Autodesk Fusion 360 part; units mm, degrees
(part 2 of 4)
  line L926 (106.594, 72.9326) -> (106.594, 69.8334)
  line L927 (106.594, 69.8334) -> (107.395, 69.8334)
  line L928 (107.395, 69.8334) -> (107.395, 64.0334)
  line L929 (107.395, 64.0334) -> (106.594, 64.0334)
  line L930 (106.594, 64.0334) -> (106.594, 60.9328)
  line L931 (106.594, 60.9328) -> (107.395, 60.9328)
  line L932 (107.395, 60.9328) -> (107.395, 59.9338)
  line L933 (107.395, 59.9338) -> (121.394, 59.9338)
  line L934 (121.394, 59.9338) -> (121.394, 60.9328)
  line L935 (121.394, 60.9328) -> (122.195, 60.9328)
  line L936 (122.195, 60.9328) -> (122.195, 64.0334)
  line L937 (122.195, 64.0334) -> (121.394, 64.0334)
  line L938 (121.394, 64.0334) -> (121.394, 69.8334)
  line L939 (121.394, 69.8334) -> (122.195, 69.8334)
  line L940 (122.195, 69.8334) -> (122.195, 72.9326)
  line L941 (122.195, 72.9326) -> (121.394, 72.9326)
  line L942 (121.394, 72.9326) -> (121.394, 73.9331)
  line L943 (121.394, 73.9331) -> (107.395, 73.9331)
  line L944 (126.445, 73.9331) -> (126.445, 72.9326)
  line L945 (126.445, 72.9326) -> (125.644, 72.9326)
  line L946 (125.644, 72.9326) -> (125.644, 69.8334)
  line L947 (125.644, 69.8334) -> (126.445, 69.8334)
  line L948 (126.445, 69.8334) -> (126.445, 64.0334)
  line L949 (126.445, 64.0334) -> (125.644, 64.0334)
  line L950 (125.644, 64.0334) -> (125.644, 60.9328)
  line L951 (125.644, 60.9328) -> (126.445, 60.9328)
  line L952 (126.445, 60.9328) -> (126.445, 59.9338)
  line L953 (126.445, 59.9338) -> (140.444, 59.9338)
  line L954 (140.444, 59.9338) -> (140.444, 60.9328)
  line L955 (140.444, 60.9328) -> (141.245, 60.9328)
  line L956 (141.245, 60.9328) -> (141.245, 64.0334)
  line L957 (141.245, 64.0334) -> (140.444, 64.0334)
  line L958 (140.444, 64.0334) -> (140.444, 69.8334)
  line L959 (140.444, 69.8334) -> (141.245, 69.8334)
  line L960 (141.245, 69.8334) -> (141.245, 72.9326)
  line L961 (141.245, 72.9326) -> (140.444, 72.9326)
  line L962 (140.444, 72.9326) -> (140.444, 73.9331)
  line L963 (140.444, 73.9331) -> (126.445, 73.9331)
  line L964 (145.495, 73.9331) -> (145.495, 72.9326)
  line L965 (145.495, 72.9326) -> (144.694, 72.9326)
  line L966 (144.694, 72.9326) -> (144.694, 69.8334)
  line L967 (144.694, 69.8334) -> (145.495, 69.8334)
  line L968 (145.495, 69.8334) -> (145.495, 64.0334)
  line L969 (145.495, 64.0334) -> (144.694, 64.0334)
  line L970 (144.694, 64.0334) -> (144.694, 60.9328)
  line L971 (144.694, 60.9328) -> (145.495, 60.9328)
  line L972 (145.495, 60.9328) -> (145.495, 59.9338)
  line L973 (145.495, 59.9338) -> (159.494, 59.9338)
  line L974 (159.494, 59.9338) -> (159.494, 60.9328)
  line L975 (159.494, 60.9328) -> (160.295, 60.9328)
  line L976 (160.295, 60.9328) -> (160.295, 64.0334)
  line L977 (160.295, 64.0334) -> (159.494, 64.0334)
  line L978 (159.494, 64.0334) -> (159.494, 69.8334)
  line L979 (159.494, 69.8334) -> (160.295, 69.8334)
  line L980 (160.295, 69.8334) -> (160.295, 72.9326)
  line L981 (160.295, 72.9326) -> (159.494, 72.9326)
  line L982 (159.494, 72.9326) -> (159.494, 73.9331)
  line L983 (159.494, 73.9331) -> (145.495, 73.9331)
  line L984 (164.545, 73.9331) -> (164.545, 72.9326)
  line L985 (164.545, 72.9326) -> (163.744, 72.9326)
  line L986 (163.744, 72.9326) -> (163.744, 69.8334)
  line L987 (163.744, 69.8334) -> (164.545, 69.8334)
  line L988 (164.545, 69.8334) -> (164.545, 64.0334)
  line L989 (164.545, 64.0334) -> (163.744, 64.0334)
  line L990 (163.744, 64.0334) -> (163.744, 60.9328)
  line L991 (163.744, 60.9328) -> (164.545, 60.9328)
  line L992 (164.545, 60.9328) -> (164.545, 59.9338)
  line L993 (164.545, 59.9338) -> (178.544, 59.9338)
  line L994 (178.544, 59.9338) -> (178.544, 60.9328)
  line L995 (178.544, 60.9328) -> (179.345, 60.9328)
  line L996 (179.345, 60.9328) -> (179.345, 64.0334)
  line L997 (179.345, 64.0334) -> (178.544, 64.0334)
  line L998 (178.544, 64.0334) -> (178.544, 69.8334)
  line L999 (178.544, 69.8334) -> (179.345, 69.8334)
  line L1000 (179.345, 69.8334) -> (179.345, 72.9326)
  line L1001 (179.345, 72.9326) -> (178.544, 72.9326)
  line L1002 (178.544, 72.9326) -> (178.544, 73.9331)
  line L1003 (178.544, 73.9331) -> (164.545, 73.9331)
  line L1004 (183.595, 73.9331) -> (183.595, 72.9326)
  line L1005 (183.595, 72.9326) -> (182.794, 72.9326)
  line L1006 (182.794, 72.9326) -> (182.794, 69.8334)
  line L1007 (182.794, 69.8334) -> (183.595, 69.8334)
  line L1008 (183.595, 69.8334) -> (183.595, 64.0334)
  line L1009 (183.595, 64.0334) -> (182.794, 64.0334)
  line L1010 (182.794, 64.0334) -> (182.794, 60.9328)
  line L1011 (182.794, 60.9328) -> (183.595, 60.9328)
  line L1012 (183.595, 60.9328) -> (183.595, 59.9338)
  line L1013 (183.595, 59.9338) -> (197.594, 59.9338)
  line L1014 (197.594, 59.9338) -> (197.594, 60.9328)
  line L1015 (197.594, 60.9328) -> (198.395, 60.9328)
  line L1016 (198.395, 60.9328) -> (198.395, 64.0334)
  line L1017 (198.395, 64.0334) -> (197.594, 64.0334)
  line L1018 (197.594, 64.0334) -> (197.594, 69.8334)
  line L1019 (197.594, 69.8334) -> (198.395, 69.8334)
  line L1020 (198.395, 69.8334) -> (198.395, 72.9326)
  line L1021 (198.395, 72.9326) -> (197.594, 72.9326)
  line L1022 (197.594, 72.9326) -> (197.594, 73.9331)
  line L1023 (197.594, 73.9331) -> (183.595, 73.9331)
  line L1024 (202.645, 73.9331) -> (202.645, 72.9326)
  line L1025 (202.645, 72.9326) -> (201.844, 72.9326)
  line L1026 (201.844, 72.9326) -> (201.844, 69.8334)
  line L1027 (201.844, 69.8334) -> (202.645, 69.8334)
  line L1028 (202.645, 69.8334) -> (202.645, 64.0334)
  line L1029 (202.645, 64.0334) -> (201.844, 64.0334)
  line L1030 (201.844, 64.0334) -> (201.844, 60.9328)
  line L1031 (201.844, 60.9328) -> (202.645, 60.9328)
  line L1032 (202.645, 60.9328) -> (202.645, 59.9338)
  line L1033 (202.645, 59.9338) -> (216.644, 59.9338)
  line L1034 (216.644, 59.9338) -> (216.644, 60.9328)
  line L1035 (216.644, 60.9328) -> (217.445, 60.9328)
  line L1036 (217.445, 60.9328) -> (217.445, 64.0334)
  line L1037 (217.445, 64.0334) -> (216.644, 64.0334)
  line L1038 (216.644, 64.0334) -> (216.644, 69.8334)
  line L1039 (216.644, 69.8334) -> (217.445, 69.8334)
  line L1040 (217.445, 69.8334) -> (217.445, 72.9326)
  line L1041 (217.445, 72.9326) -> (216.644, 72.9326)
  line L1042 (216.644, 72.9326) -> (216.644, 73.9331)
  line L1043 (216.644, 73.9331) -> (202.645, 73.9331)
  line L1044 (221.695, 73.9331) -> (221.695, 72.9326)
  line L1045 (221.695, 72.9326) -> (220.894, 72.9326)
  line L1046 (220.894, 72.9326) -> (220.894, 69.8334)
  line L1047 (220.894, 69.8334) -> (221.695, 69.8334)
  line L1048 (221.695, 69.8334) -> (221.695, 64.0334)
  line L1049 (221.695, 64.0334) -> (220.894, 64.0334)
  line L1050 (220.894, 64.0334) -> (220.894, 60.9328)
  line L1051 (220.894, 60.9328) -> (221.695, 60.9328)
  line L1052 (221.695, 60.9328) -> (221.695, 59.9338)
  line L1053 (221.695, 59.9338) -> (235.694, 59.9338)
  line L1054 (235.694, 59.9338) -> (235.694, 60.9328)
  line L1055 (235.694, 60.9328) -> (236.495, 60.9328)
  line L1056 (236.495, 60.9328) -> (236.495, 64.0334)
  line L1057 (236.495, 64.0334) -> (235.694, 64.0334)
  line L1058 (235.694, 64.0334) -> (235.694, 69.8334)
  line L1059 (235.694, 69.8334) -> (236.495, 69.8334)
  line L1060 (236.495, 69.8334) -> (236.495, 72.9326)
  line L1061 (236.495, 72.9326) -> (235.694, 72.9326)
  line L1062 (235.694, 72.9326) -> (235.694, 73.9331)
  line L1063 (235.694, 73.9331) -> (221.695, 73.9331)
  line L1064 (240.745, 73.9331) -> (240.745, 72.9326)
  line L1065 (240.745, 72.9326) -> (239.944, 72.9326)
  line L1066 (239.944, 72.9326) -> (239.944, 69.8334)
  line L1067 (239.944, 69.8334) -> (240.745, 69.8334)
  line L1068 (240.745, 69.8334) -> (240.745, 64.0334)
  line L1069 (240.745, 64.0334) -> (239.944, 64.0334)
  line L1070 (239.944, 64.0334) -> (239.944, 60.9328)
  line L1071 (239.944, 60.9328) -> (240.745, 60.9328)
  line L1072 (240.745, 60.9328) -> (240.745, 59.9338)
  line L1073 (240.745, 59.9338) -> (254.744, 59.9338)
  line L1074 (254.744, 59.9338) -> (254.744, 60.9328)
  line L1075 (254.744, 60.9328) -> (255.545, 60.9328)
  line L1076 (255.545, 60.9328) -> (255.545, 64.0334)
  line L1077 (255.545, 64.0334) -> (254.744, 64.0334)
  line L1078 (254.744, 64.0334) -> (254.744, 69.8334)
  line L1079 (254.744, 69.8334) -> (255.545, 69.8334)
  line L1080 (255.545, 69.8334) -> (255.545, 72.9326)
  line L1081 (255.545, 72.9326) -> (254.744, 72.9326)
  line L1082 (254.744, 72.9326) -> (254.744, 73.9331)
  line L1083 (254.744, 73.9331) -> (240.745, 73.9331)
  line L1084 (264.557, 73.9331) -> (264.557, 72.9326)
  line L1085 (264.557, 72.9326) -> (263.756, 72.9326)
  line L1086 (263.756, 72.9326) -> (263.756, 69.8334)
  line L1087 (263.756, 69.8334) -> (264.557, 69.8334)
  line L1088 (264.557, 69.8334) -> (264.557, 64.0334)
  line L1089 (264.557, 64.0334) -> (263.756, 64.0334)
  line L1090 (263.756, 64.0334) -> (263.756, 60.9328)
  line L1091 (263.756, 60.9328) -> (264.557, 60.9328)
  line L1092 (264.557, 60.9328) -> (264.557, 59.9338)
  line L1093 (264.557, 59.9338) -> (278.557, 59.9338)
  line L1094 (278.557, 59.9338) -> (278.557, 60.9328)
  line L1095 (278.557, 60.9328) -> (279.356, 60.9328)
  line L1096 (279.356, 60.9328) -> (279.356, 64.0334)
  line L1097 (279.356, 64.0334) -> (278.557, 64.0334)
  line L1098 (278.557, 64.0334) -> (278.557, 69.8334)
  line L1099 (278.557, 69.8334) -> (279.356, 69.8334)
  line L1100 (279.356, 69.8334) -> (279.356, 72.9326)
  line L1101 (279.356, 72.9326) -> (278.557, 72.9326)
  line L1102 (278.557, 72.9326) -> (278.557, 73.9331)
  line L1103 (278.557, 73.9331) -> (264.557, 73.9331)
  line L1104 (259.795, 92.9831) -> (259.795, 91.9826)
  line L1105 (259.795, 91.9826) -> (258.994, 91.9826)
  line L1106 (258.994, 91.9826) -> (258.994, 88.8834)
  line L1107 (258.994, 88.8834) -> (259.795, 88.8834)
  line L1108 (259.795, 88.8834) -> (259.795, 88.2826)
  line L1109 (259.795, 88.2826) -> (258.269, 88.2826)
  line L1110 (258.269, 88.2826) -> (258.269, 91.5127)
  line L1111 (258.269, 91.5127) -> (256.544, 91.5127)
  line L1112 (256.544, 91.5127) -> (256.544, 92.4348)
  line L1113 (256.544, 92.4348) -> (253.243, 92.4348)
  line L1114 (253.243, 92.4348) -> (253.243, 91.5127)
  line L1115 (253.243, 91.5127) -> (251.52, 91.5127)
  line L1116 (251.52, 91.5127) -> (251.52, 88.2826)
  line L1117 (251.52, 88.2826) -> (250.694, 88.2826)
  line L1118 (250.694, 88.2826) -> (250.694, 85.4837)
  line L1119 (250.694, 85.4837) -> (251.52, 85.4837)
  line L1120 (251.52, 85.4837) -> (251.52, 79.2138)
  line L1121 (251.52, 79.2138) -> (253.243, 79.2138)
  line L1122 (253.243, 79.2138) -> (253.243, 78.2327)
  line L1123 (253.243, 78.2327) -> (256.544, 78.2327)
  line L1124 (256.544, 78.2327) -> (256.544, 79.2138)
  line L1125 (256.544, 79.2138) -> (258.269, 79.2138)
  line L1126 (258.269, 79.2138) -> (258.269, 83.6828)
  line L1127 (258.269, 83.6828) -> (259.795, 83.6828)
  line L1128 (259.795, 83.6828) -> (259.795, 83.0834)
  line L1129 (259.795, 83.0834) -> (258.994, 83.0834)
  line L1130 (258.994, 83.0834) -> (258.994, 79.9828)
  line L1131 (258.994, 79.9828) -> (259.795, 79.9828)
  line L1132 (259.795, 79.9828) -> (259.795, 78.9838)
  line L1133 (259.795, 78.9838) -> (273.794, 78.9838)
  line L1134 (273.794, 78.9838) -> (273.794, 79.9828)
  line L1135 (273.794, 79.9828) -> (274.595, 79.9828)
  line L1136 (274.595, 79.9828) -> (274.595, 83.0834)
  line L1137 (274.595, 83.0834) -> (273.794, 83.0834)
  line L1138 (273.794, 83.0834) -> (273.794, 83.6828)
  line L1139 (273.794, 83.6828) -> (275.32, 83.6828)
  line L1140 (275.32, 83.6828) -> (275.32, 79.2138)
  line L1141 (275.32, 79.2138) -> (277.045, 79.2138)
  line L1142 (277.045, 79.2138) -> (277.045, 78.2327)
  line L1143 (277.045, 78.2327) -> (280.344, 78.2327)
  line L1144 (280.344, 78.2327) -> (280.344, 79.2138)
  line L1145 (280.344, 79.2138) -> (282.069, 79.2138)
  line L1146 (282.069, 79.2138) -> (282.069, 85.4837)
  line L1147 (282.069, 85.4837) -> (282.895, 85.4837)
  line L1148 (282.895, 85.4837) -> (282.895, 88.2826)
  line L1149 (282.895, 88.2826) -> (282.069, 88.2826)
  line L1150 (282.069, 88.2826) -> (282.069, 91.5127)
  line L1151 (282.069, 91.5127) -> (280.344, 91.5127)
  line L1152 (280.344, 91.5127) -> (280.344, 92.4348)
  line L1153 (280.344, 92.4348) -> (277.045, 92.4348)
  line L1154 (277.045, 92.4348) -> (277.045, 91.5127)
  line L1155 (277.045, 91.5127) -> (275.32, 91.5127)
  line L1156 (275.32, 91.5127) -> (275.32, 88.2826)
  line L1157 (275.32, 88.2826) -> (273.794, 88.2826)
  line L1158 (273.794, 88.2826) -> (273.794, 88.8834)
  line L1159 (273.794, 88.8834) -> (274.595, 88.8834)
  line L1160 (274.595, 88.8834) -> (274.595, 91.9826)
  line L1161 (274.595, 91.9826) -> (273.794, 91.9826)
  line L1162 (273.794, 91.9826) -> (273.794, 92.9831)
  line L1163 (273.794, 92.9831) -> (259.795, 92.9831)
  line L1164 (2.6197, 92.9831) -> (2.6197, 91.9826)
  line L1165 (2.6197, 91.9826) -> (1.819, 91.9826)
  line L1166 (1.819, 91.9826) -> (1.819, 88.8834)
  line L1167 (1.819, 88.8834) -> (2.6197, 88.8834)
  line L1168 (2.6197, 88.8834) -> (2.6197, 83.0834)
  line L1169 (2.6197, 83.0834) -> (1.819, 83.0834)
  line L1170 (1.819, 83.0834) -> (1.819, 79.9828)
  line L1171 (1.819, 79.9828) -> (2.6197, 79.9828)
  line L1172 (2.6197, 79.9828) -> (2.6197, 78.9838)
  line L1173 (2.6197, 78.9838) -> (16.6192, 78.9838)
  line L1174 (16.6192, 78.9838) -> (16.6192, 79.9828)
  line L1175 (16.6192, 79.9828) -> (17.4198, 79.9828)
  line L1176 (17.4198, 79.9828) -> (17.4198, 83.0834)
  line L1177 (17.4198, 83.0834) -> (16.6192, 83.0834)
  line L1178 (16.6192, 83.0834) -> (16.6192, 88.8834)
  line L1179 (16.6192, 88.8834) -> (17.4198, 88.8834)
  line L1180 (17.4198, 88.8834) -> (17.4198, 91.9826)
  line L1181 (17.4198, 91.9826) -> (16.6192, 91.9826)
  line L1182 (16.6192, 91.9826) -> (16.6192, 92.9831)
  line L1183 (16.6192, 92.9831) -> (2.6196, 92.9831)
  line L1184 (21.6697, 92.9831) -> (21.6697, 91.9826)
  line L1185 (21.6697, 91.9826) -> (20.869, 91.9826)
  line L1186 (20.869, 91.9826) -> (20.869, 88.8834)
  line L1187 (20.869, 88.8834) -> (21.6697, 88.8834)
  line L1188 (21.6697, 88.8834) -> (21.6697, 83.0834)
  line L1189 (21.6697, 83.0834) -> (20.869, 83.0834)
  line L1190 (20.869, 83.0834) -> (20.869, 79.9828)
  line L1191 (20.869, 79.9828) -> (21.6697, 79.9828)
  line L1192 (21.6697, 79.9828) -> (21.6697, 78.9838)
  line L1193 (21.6697, 78.9838) -> (35.669, 78.9838)
  line L1194 (35.669, 78.9838) -> (35.669, 79.9828)
  line L1195 (35.669, 79.9828) -> (36.4698, 79.9828)
  line L1196 (36.4698, 79.9828) -> (36.4698, 83.0834)
  line L1197 (36.4698, 83.0834) -> (35.669, 83.0834)
  line L1198 (35.669, 83.0834) -> (35.669, 88.8834)
  line L1199 (35.669, 88.8834) -> (36.4698, 88.8834)
  line L1200 (36.4698, 88.8834) -> (36.4698, 91.9826)
  line L1201 (36.4698, 91.9826) -> (35.669, 91.9826)
  line L1202 (35.669, 91.9826) -> (35.669, 92.9831)
  line L1203 (35.669, 92.9831) -> (21.6697, 92.9831)
  line L1204 (40.7197, 92.9831) -> (40.7197, 91.9826)
  line L1205 (40.7197, 91.9826) -> (39.9189, 91.9826)
  line L1206 (39.9189, 91.9826) -> (39.9189, 88.8834)
  line L1207 (39.9189, 88.8834) -> (40.7197, 88.8834)
  line L1208 (40.7197, 88.8834) -> (40.7197, 83.0834)
  line L1209 (40.7197, 83.0834) -> (39.9189, 83.0834)
  line L1210 (39.9189, 83.0834) -> (39.9189, 79.9828)
  line L1211 (39.9189, 79.9828) -> (40.7197, 79.9828)
  line L1212 (40.7197, 79.9828) -> (40.7197, 78.9838)
  line L1213 (40.7197, 78.9838) -> (54.719, 78.9838)
  line L1214 (54.719, 78.9838) -> (54.719, 79.9828)
  line L1215 (54.719, 79.9828) -> (55.5198, 79.9828)
  line L1216 (55.5198, 79.9828) -> (55.5198, 83.0834)
  line L1217 (55.5198, 83.0834) -> (54.719, 83.0834)
  line L1218 (54.719, 83.0834) -> (54.719, 88.8834)
  line L1219 (54.719, 88.8834) -> (55.5198, 88.8834)
  line L1220 (55.5198, 88.8834) -> (55.5198, 91.9826)
  line L1221 (55.5198, 91.9826) -> (54.719, 91.9826)
  line L1222 (54.719, 91.9826) -> (54.719, 92.9831)
  line L1223 (54.719, 92.9831) -> (40.7197, 92.9831)
  line L1224 (59.7697, 92.9831) -> (59.7697, 91.9826)
  line L1225 (59.7697, 91.9826) -> (58.9689, 91.9826)
  line L1226 (58.9689, 91.9826) -> (58.9689, 88.8834)
  line L1227 (58.9689, 88.8834) -> (59.7697, 88.8834)
  line L1228 (59.7697, 88.8834) -> (59.7697, 83.0834)
  line L1229 (59.7697, 83.0834) -> (58.9689, 83.0834)
  line L1230 (58.9689, 83.0834) -> (58.9689, 79.9828)
  line L1231 (58.9689, 79.9828) -> (59.7697, 79.9828)
  line L1232 (59.7697, 79.9828) -> (59.7697, 78.9838)
  line L1233 (59.7697, 78.9838) -> (73.769, 78.9838)
  line L1234 (73.769, 78.9838) -> (73.769, 79.9828)
  line L1235 (73.769, 79.9828) -> (74.5698, 79.9828)
  line L1236 (74.5698, 79.9828) -> (74.5698, 83.0834)
  line L1237 (74.5698, 83.0834) -> (73.769, 83.0834)
  line L1238 (73.769, 83.0834) -> (73.769, 88.8834)
  line L1239 (73.769, 88.8834) -> (74.5698, 88.8834)
  line L1240 (74.5698, 88.8834) -> (74.5698, 91.9826)
  line L1241 (74.5698, 91.9826) -> (73.769, 91.9826)
  line L1242 (73.769, 91.9826) -> (73.769, 92.9831)
  line L1243 (73.769, 92.9831) -> (59.7697, 92.9831)
  line L1244 (78.8197, 92.9831) -> (78.8197, 91.9826)
  line L1245 (78.8197, 91.9826) -> (78.0189, 91.9826)
  line L1246 (78.0189, 91.9826) -> (78.0189, 88.8834)
  line L1247 (78.0189, 88.8834) -> (78.8197, 88.8834)
  line L1248 (78.8197, 88.8834) -> (78.8197, 83.0834)
  line L1249 (78.8197, 83.0834) -> (78.0189, 83.0834)
  line L1250 (78.0189, 83.0834) -> (78.0189, 79.9828)
  line L1251 (78.0189, 79.9828) -> (78.8197, 79.9828)
  line L1252 (78.8197, 79.9828) -> (78.8197, 78.9838)
  line L1253 (78.8197, 78.9838) -> (92.819, 78.9838)
  line L1254 (92.819, 78.9838) -> (92.819, 79.9828)
  line L1255 (92.819, 79.9828) -> (93.6184, 79.9828)
  line L1256 (93.6184, 79.9828) -> (93.6184, 83.0834)
  line L1257 (93.6184, 83.0834) -> (92.819, 83.0834)
  line L1258 (92.819, 83.0834) -> (92.819, 88.8834)
  line L1259 (92.819, 88.8834) -> (93.6184, 88.8834)
  line L1260 (93.6184, 88.8834) -> (93.6184, 91.9826)
  line L1261 (93.6184, 91.9826) -> (92.819, 91.9826)
  line L1262 (92.819, 91.9826) -> (92.819, 92.9831)
  line L1263 (92.819, 92.9831) -> (78.8197, 92.9831)
  line L1264 (97.8683, 92.9831) -> (97.8683, 91.9826)
  line L1265 (97.8683, 91.9826) -> (97.0689, 91.9826)
  line L1266 (97.0689, 91.9826) -> (97.0689, 88.8834)
  line L1267 (97.0689, 88.8834) -> (97.8683, 88.8834)
  line L1268 (97.8683, 88.8834) -> (97.8683, 83.0834)
  line L1269 (97.8683, 83.0834) -> (97.0689, 83.0834)
  line L1270 (97.0689, 83.0834) -> (97.0689, 79.9828)
  line L1271 (97.0689, 79.9828) -> (97.8683, 79.9828)
  line L1272 (97.8683, 79.9828) -> (97.8683, 78.9838)
  line L1273 (97.8683, 78.9838) -> (111.869, 78.9838)
  line L1274 (111.869, 78.9838) -> (111.869, 79.9828)
  line L1275 (111.869, 79.9828) -> (112.668, 79.9828)
  line L1276 (112.668, 79.9828) -> (112.668, 83.0834)
  line L1277 (112.668, 83.0834) -> (111.869, 83.0834)
  line L1278 (111.869, 83.0834) -> (111.869, 88.8834)
  line L1279 (111.869, 88.8834) -> (112.668, 88.8834)
  line L1280 (112.668, 88.8834) -> (112.668, 91.9826)
  line L1281 (112.668, 91.9826) -> (111.869, 91.9826)
  line L1282 (111.869, 91.9826) -> (111.869, 92.9831)
  line L1283 (111.869, 92.9831) -> (97.8683, 92.9831)
  line L1284 (116.918, 92.9831) -> (116.918, 91.9826)
  line L1285 (116.918, 91.9826) -> (116.119, 91.9826)
  line L1286 (116.119, 91.9826) -> (116.119, 88.8834)
  line L1287 (116.119, 88.8834) -> (116.918, 88.8834)
  line L1288 (116.918, 88.8834) -> (116.918, 83.0834)
  line L1289 (116.918, 83.0834) -> (116.119, 83.0834)
  line L1290 (116.119, 83.0834) -> (116.119, 79.9828)
  line L1291 (116.119, 79.9828) -> (116.918, 79.9828)
  line L1292 (116.918, 79.9828) -> (116.918, 78.9838)
  line L1293 (116.918, 78.9838) -> (130.919, 78.9838)
  line L1294 (130.919, 78.9838) -> (130.919, 79.9828)
  line L1295 (130.919, 79.9828) -> (131.72, 79.9828)
  line L1296 (131.72, 79.9828) -> (131.72, 83.0834)
  line L1297 (131.72, 83.0834) -> (130.919, 83.0834)
  line L1298 (130.919, 83.0834) -> (130.919, 88.8834)
  line L1299 (130.919, 88.8834) -> (131.72, 88.8834)
  line L1300 (131.72, 88.8834) -> (131.72, 91.9826)
  line L1301 (131.72, 91.9826) -> (130.919, 91.9826)
  line L1302 (130.919, 91.9826) -> (130.919, 92.9831)
  line L1303 (130.919, 92.9831) -> (116.918, 92.9831)
  line L1304 (135.97, 92.9831) -> (135.97, 91.9826)
  line L1305 (135.97, 91.9826) -> (135.169, 91.9826)
  line L1306 (135.169, 91.9826) -> (135.169, 88.8834)
  line L1307 (135.169, 88.8834) -> (135.97, 88.8834)
  line L1308 (135.97, 88.8834) -> (135.97, 83.0834)
  line L1309 (135.97, 83.0834) -> (135.169, 83.0834)
  line L1310 (135.169, 83.0834) -> (135.169, 79.9828)
  line L1311 (135.169, 79.9828) -> (135.97, 79.9828)
  line L1312 (135.97, 79.9828) -> (135.97, 78.9838)
  line L1313 (135.97, 78.9838) -> (149.969, 78.9838)
  line L1314 (149.969, 78.9838) -> (149.969, 79.9828)
  line L1315 (149.969, 79.9828) -> (150.77, 79.9828)
  line L1316 (150.77, 79.9828) -> (150.77, 83.0834)
  line L1317 (150.77, 83.0834) -> (149.969, 83.0834)
  line L1318 (149.969, 83.0834) -> (149.969, 88.8834)
  line L1319 (149.969, 88.8834) -> (150.77, 88.8834)
  line L1320 (150.77, 88.8834) -> (150.77, 91.9826)
  line L1321 (150.77, 91.9826) -> (149.969, 91.9826)
  line L1322 (149.969, 91.9826) -> (149.969, 92.9831)
  line L1323 (149.969, 92.9831) -> (135.97, 92.9831)
  line L1324 (155.02, 92.9831) -> (155.02, 91.9826)
  line L1325 (155.02, 91.9826) -> (154.219, 91.9826)
  line L1326 (154.219, 91.9826) -> (154.219, 88.8834)
  line L1327 (154.219, 88.8834) -> (155.02, 88.8834)
  line L1328 (155.02, 88.8834) -> (155.02, 83.0834)
  line L1329 (155.02, 83.0834) -> (154.219, 83.0834)
  line L1330 (154.219, 83.0834) -> (154.219, 79.9828)
  line L1331 (154.219, 79.9828) -> (155.02, 79.9828)
  line L1332 (155.02, 79.9828) -> (155.02, 78.9838)
  line L1333 (155.02, 78.9838) -> (169.019, 78.9838)
  line L1334 (169.019, 78.9838) -> (169.019, 79.9828)
  line L1335 (169.019, 79.9828) -> (169.82, 79.9828)
  line L1336 (169.82, 79.9828) -> (169.82, 83.0834)
  line L1337 (169.82, 83.0834) -> (169.019, 83.0834)
  line L1338 (169.019, 83.0834) -> (169.019, 88.8834)
  line L1339 (169.019, 88.8834) -> (169.82, 88.8834)
  line L1340 (169.82, 88.8834) -> (169.82, 91.9826)
  line L1341 (169.82, 91.9826) -> (169.019, 91.9826)
  line L1342 (169.019, 91.9826) -> (169.019, 92.9831)
  line L1343 (169.019, 92.9831) -> (155.02, 92.9831)
  line L1344 (174.07, 92.9831) -> (174.07, 91.9826)
  line L1345 (174.07, 91.9826) -> (173.269, 91.9826)
  line L1346 (173.269, 91.9826) -> (173.269, 88.8834)
  line L1347 (173.269, 88.8834) -> (174.07, 88.8834)
  line L1348 (174.07, 88.8834) -> (174.07, 83.0834)
  line L1349 (174.07, 83.0834) -> (173.269, 83.0834)
  line L1350 (173.269, 83.0834) -> (173.269, 79.9828)
  line L1351 (173.269, 79.9828) -> (174.07, 79.9828)
  line L1352 (174.07, 79.9828) -> (174.07, 78.9838)
  line L1353 (174.07, 78.9838) -> (188.069, 78.9838)
  line L1354 (188.069, 78.9838) -> (188.069, 79.9828)
  line L1355 (188.069, 79.9828) -> (188.87, 79.9828)
  line L1356 (188.87, 79.9828) -> (188.87, 83.0834)
  line L1357 (188.87, 83.0834) -> (188.069, 83.0834)
  line L1358 (188.069, 83.0834) -> (188.069, 88.8834)
  line L1359 (188.069, 88.8834) -> (188.87, 88.8834)
  line L1360 (188.87, 88.8834) -> (188.87, 91.9826)
  line L1361 (188.87, 91.9826) -> (188.069, 91.9826)
  line L1362 (188.069, 91.9826) -> (188.069, 92.9831)
  line L1363 (188.069, 92.9831) -> (174.07, 92.9831)
  line L1364 (193.12, 92.9831) -> (193.12, 91.9826)
  line L1365 (193.12, 91.9826) -> (192.319, 91.9826)
  line L1366 (192.319, 91.9826) -> (192.319, 88.8834)
  line L1367 (192.319, 88.8834) -> (193.12, 88.8834)
  line L1368 (193.12, 88.8834) -> (193.12, 83.0834)
  line L1369 (193.12, 83.0834) -> (192.319, 83.0834)
  line L1370 (192.319, 83.0834) -> (192.319, 79.9828)
  line L1371 (192.319, 79.9828) -> (193.12, 79.9828)
  line L1372 (193.12, 79.9828) -> (193.12, 78.9838)
  line L1373 (193.12, 78.9838) -> (207.119, 78.9838)
  line L1374 (207.119, 78.9838) -> (207.119, 79.9828)
  line L1375 (207.119, 79.9828) -> (207.92, 79.9828)
  line L1376 (207.92, 79.9828) -> (207.92, 83.0834)
  line L1377 (207.92, 83.0834) -> (207.119, 83.0834)
  line L1378 (207.119, 83.0834) -> (207.119, 88.8834)
  line L1379 (207.119, 88.8834) -> (207.92, 88.8834)
  line L1380 (207.92, 88.8834) -> (207.92, 91.9826)
  line L1381 (207.92, 91.9826) -> (207.119, 91.9826)
  line L1382 (207.119, 91.9826) -> (207.119, 92.9831)
  line L1383 (207.119, 92.9831) -> (193.12, 92.9831)
  line L1384 (212.17, 92.9831) -> (212.17, 91.9826)
  line L1385 (212.17, 91.9826) -> (211.369, 91.9826)
  line L1386 (211.369, 91.9826) -> (211.369, 88.8834)
  line L1387 (211.369, 88.8834) -> (212.17, 88.8834)
  line L1388 (212.17, 88.8834) -> (212.17, 83.0834)
  line L1389 (212.17, 83.0834) -> (211.369, 83.0834)
  line L1390 (211.369, 83.0834) -> (211.369, 79.9828)
  line L1391 (211.369, 79.9828) -> (212.17, 79.9828)
  line L1392 (212.17, 79.9828) -> (212.17, 78.9838)
  line L1393 (212.17, 78.9838) -> (226.169, 78.9838)
  line L1394 (226.169, 78.9838) -> (226.169, 79.9828)
  line L1395 (226.169, 79.9828) -> (226.97, 79.9828)
  line L1396 (226.97, 79.9828) -> (226.97, 83.0834)
  line L1397 (226.97, 83.0834) -> (226.169, 83.0834)
  line L1398 (226.169, 83.0834) -> (226.169, 88.8834)
  line L1399 (226.169, 88.8834) -> (226.97, 88.8834)
  line L1400 (226.97, 88.8834) -> (226.97, 91.9826)
  line L1401 (226.97, 91.9826) -> (226.169, 91.9826)
  line L1402 (226.169, 91.9826) -> (226.169, 92.9831)
  line L1403 (226.169, 92.9831) -> (212.17, 92.9831)
  line L1404 (231.22, 92.9831) -> (231.22, 91.9826)
  line L1405 (231.22, 91.9826) -> (230.419, 91.9826)
  line L1406 (230.419, 91.9826) -> (230.419, 88.8834)
  line L1407 (230.419, 88.8834) -> (231.22, 88.8834)
  line L1408 (231.22, 88.8834) -> (231.22, 83.0834)
  line L1409 (231.22, 83.0834) -> (230.419, 83.0834)
  line L1410 (230.419, 83.0834) -> (230.419, 79.9828)
  line L1411 (230.419, 79.9828) -> (231.22, 79.9828)
  line L1412 (231.22, 79.9828) -> (231.22, 78.9838)
  line L1413 (231.22, 78.9838) -> (245.219, 78.9838)
  line L1414 (245.219, 78.9838) -> (245.219, 79.9828)
  line L1415 (245.219, 79.9828) -> (246.02, 79.9828)
  line L1416 (246.02, 79.9828) -> (246.02, 83.0834)
  line L1417 (246.02, 83.0834) -> (245.219, 83.0834)
  line L1418 (245.219, 83.0834) -> (245.219, 88.8834)
  line L1419 (245.219, 88.8834) -> (246.02, 88.8834)
  line L1420 (246.02, 88.8834) -> (246.02, 91.9826)
  line L1421 (246.02, 91.9826) -> (245.219, 91.9826)
  line L1422 (245.219, 91.9826) -> (245.219, 92.9831)
  line L1423 (245.219, 92.9831) -> (231.22, 92.9831)
extrude "Extrude3" add sketch "48cd8e48e3c34c88b59e201f8eb7611360cf066c_switch" along normal blind 1.6 separate body makes body 2
move_body "Move1" bodies 2 to x (1, 0, 0) y (0, 1, 0) z (0, 0, 1) at (15, 9, -15)
extrude "Extrude4" add 1 faces at (205.595, 10.0667, -15.2577) along direction (0, 0, 1) blind 3 on bodies 2 bodies 2
extrude "Extrude5" add 1 faces at (205.595, 10.0667, -12.2577) along direction (0, 0, 1) blind 9 on bodies 2 bodies 2
extrude "Extrude6" add 1 faces at (15.0951, 9.5333, -74.7576) along direction (-1, 0, 0) blind 7 on bodies 2 bodies 2
extrude "Extrude7" add 1 faces at (105.6784, 9.5333, -3.2577) along direction (0, 0, 1) blind 1.3 on bodies 2 bodies 2
extrude "Extrude8" add 1 faces at (8.0951, 10.0667, -38.141) along direction (-1, 0, 0) blind 6.093 on bodies 2 bodies 2
fillet "Fillet7" radius 10 1 edges at (2.0021, 9.8, -1.9577) on bodies 2
extrude "Extrude9" add 1 faces at (201.2307, 9.5333, -110.5075) along direction (0, 0, -1) blind 38.45 on bodies 2 bodies 2
fillet "Fillet8" radius 10 1 edges at (2.0021, 9.8, -148.9575) on bodies 2
extrude "Extrude10" add 1 faces at (300.845, 9.5333, -50.9576) along direction (1, 0, 0) blind 7.1 on bodies 2 bodies 2
fillet "Fillet9" radius 10 1 edges at (307.945, 9.8, -1.9577) on bodies 2
fillet "Fillet10" radius 10 1 edges at (307.945, 9.8, -148.9575) on bodies 2
fillet "Fillet11" radius 3 8 edges at (2.9289, 14, -2.9289) (155, 14, 0) (307.0711, 14, -2.9289) (310, 14, -75.4964) (307.0711, 14, -148.0638) (155, 14, -150.9928) (2.9289, 14, -148.0638) (0, 14, -75.4964) on bodies 1
fillet "Fillet12" radius 0.5 16 edges at (307.9403, 14, -10.9088) (305.0711, 14, -4.9289) (299.0912, 14, -2.0597) (155, 14, -2) (10.9088, 14, -2.0597) (4.9289, 14, -4.9289) (2.0597, 14, -10.9088) (2, 14, -75.4964) (2.0597, 14, -140.0839) (4.9289, 14, -146.0638) (10.9088, 14, -148.9331) (155, 14, -148.9928) (299.0912, 14, -148.9331) (305.0711, 14, -146.0638) (307.9403, 14, -140.0839) (308, 14, -75.4964) on bodies 1
sketch "Sketch3" plane through (0, 0, 0) normal (-1, 0, 0) x (0, 0, 1)
  spline S0 degree 3 poles (-140.9928, 11.1033) (-140.3266, 11.1422) (-139.6599, 11.1716) (-138.9928, 11.1716) knots 4.126797 4.126797 4.126797 4.126797 4.326935 4.326935 4.326935 4.326935
  line L0 (-140.9928, 11.1033) -> (-140.9928, 0)
  line L1 (-140.9928, 0) -> (-10, 0)
  line L2 (-10, 0) -> (-10, 11.1033)
  spline S1 degree 3 poles (-12, 11.1716) (-11.333, 11.1716) (-10.666, 11.1422) (-10, 11.1033) knots 4.127933 4.127933 4.127933 4.127933 4.32807 4.32807 4.32807 4.32807
  line L3 (-12, 11.1716) -> (-138.9928, 11.1716)
  line L4 (-129.2, 9.2) -> (-129.2, 7.5)
  line L5 (-129.2, 7.5) -> (-128, 6.2)
  line L6 (-128, 6.2) -> (-122.3, 6.2)
  line L7 (-122.3, 6.2) -> (-121.1, 7.6)
  line L8 (-121.1, 7.6) -> (-121.1, 9.2)
  line L9 (-121.1, 9.2) -> (-129.2, 9.2)
  constraint perpendicular L3 L4
  constraint horizontal L6
  constraint perpendicular L6 L8
  constraint perpendicular L4 L9
extrude "Extrude11" cut sketch "Sketch3" against normal blind 11 contours L4 L5 L6 L7 L8 L9 bodies 1
sketch "Sketch4" plane through (0, 10.6, 0) normal (0, 1, 0) x (-1, 0, 0)
  arc A0 (-307.945, -138.9575) -> (-297.945, -148.9575) centre (-297.945, -138.9575) ccw
  line L0 (-297.945, -148.9575) -> (-12.0021, -148.9575)
  arc A1 (-12.0021, -148.9575) -> (-2.0021, -138.9575) centre (-12.0021, -138.9575) ccw
  line L1 (-2.0021, -138.9575) -> (-2.0021, -11.9577)
  arc A2 (-2.0021, -11.9577) -> (-12.0021, -1.9577) centre (-12.0021, -11.9577) ccw
  line L2 (-12.0021, -1.9577) -> (-297.945, -1.9577)
  arc A3 (-297.945, -1.9577) -> (-307.945, -11.9577) centre (-297.945, -11.9577) ccw
  line L3 (-307.945, -11.9577) -> (-307.945, -138.9575)
  line L4 (-236.695, -88.9331) -> (-250.694, -88.9331)
  line L5 (-250.694, -88.9331) -> (-250.694, -87.9326)
  line L6 (-250.694, -87.9326) -> (-251.495, -87.9326)
  line L7 (-251.495, -87.9326) -> (-251.495, -84.8334)
  line L8 (-251.495, -84.8334) -> (-250.694, -84.8334)
  line L9 (-250.694, -84.8334) -> (-250.694, -79.0334)
  line L10 (-250.694, -79.0334) -> (-251.495, -79.0334)
  line L11 (-251.495, -79.0334) -> (-251.495, -75.9328)
  line L12 (-251.495, -75.9328) -> (-250.694, -75.9328)
  line L13 (-250.694, -75.9328) -> (-250.694, -74.9338)
  line L14 (-250.694, -74.9338) -> (-236.695, -74.9338)
  line L15 (-236.695, -74.9338) -> (-236.695, -75.9328)
  line L16 (-236.695, -75.9328) -> (-235.894, -75.9328)
  line L17 (-235.894, -75.9328) -> (-235.894, -79.0334)
  line L18 (-235.894, -79.0334) -> (-236.695, -79.0334)
  line L19 (-236.695, -79.0334) -> (-236.695, -84.8334)
  line L20 (-236.695, -84.8334) -> (-235.894, -84.8334)
  line L21 (-235.894, -84.8334) -> (-235.894, -87.9326)
  line L22 (-235.894, -87.9326) -> (-236.695, -87.9326)
  line L23 (-236.695, -87.9326) -> (-236.695, -88.9331)
  line L24 (-255.745, -88.9331) -> (-269.744, -88.9331)
  line L25 (-269.744, -88.9331) -> (-269.744, -87.9326)
  line L26 (-269.744, -87.9326) -> (-270.545, -87.9326)
  line L27 (-270.545, -87.9326) -> (-270.545, -84.8334)
  line L28 (-270.545, -84.8334) -> (-269.744, -84.8334)
  line L29 (-269.744, -84.8334) -> (-269.744, -79.0334)
  line L30 (-269.744, -79.0334) -> (-270.545, -79.0334)
  line L31 (-270.545, -79.0334) -> (-270.545, -75.9328)
  line L32 (-270.545, -75.9328) -> (-269.744, -75.9328)
  line L33 (-269.744, -75.9328) -> (-269.744, -74.9338)
  line L34 (-269.744, -74.9338) -> (-255.745, -74.9338)
  line L35 (-255.745, -74.9338) -> (-255.745, -75.9328)
  line L36 (-255.745, -75.9328) -> (-254.944, -75.9328)
  line L37 (-254.944, -75.9328) -> (-254.944, -79.0334)
  line L38 (-254.944, -79.0334) -> (-255.745, -79.0334)
  line L39 (-255.745, -79.0334) -> (-255.745, -84.8334)
  line L40 (-255.745, -84.8334) -> (-254.944, -84.8334)
  line L41 (-254.944, -84.8334) -> (-254.944, -87.9326)
  line L42 (-254.944, -87.9326) -> (-255.745, -87.9326)
  line L43 (-255.745, -87.9326) -> (-255.745, -88.9331)
  line L44 (-112.8683, -107.9831) -> (-126.869, -107.9831)
  line L45 (-126.869, -107.9831) -> (-126.869, -106.9826)
  line L46 (-126.869, -106.9826) -> (-127.668, -106.9826)
  line L47 (-127.668, -106.9826) -> (-127.668, -103.8834)
  line L48 (-127.668, -103.8834) -> (-126.869, -103.8834)
  line L49 (-126.869, -103.8834) -> (-126.869, -98.0834)
  line L50 (-126.869, -98.0834) -> (-127.668, -98.0834)
  line L51 (-127.668, -98.0834) -> (-127.668, -94.9828)
  line L52 (-127.668, -94.9828) -> (-126.869, -94.9828)
  line L53 (-126.869, -94.9828) -> (-126.869, -93.9838)
  line L54 (-126.869, -93.9838) -> (-112.8683, -93.9838)
  line L55 (-112.8683, -93.9838) -> (-112.8683, -94.9828)
  line L56 (-112.8683, -94.9828) -> (-112.0689, -94.9828)
  line L57 (-112.0689, -94.9828) -> (-112.0689, -98.0834)
  line L58 (-112.0689, -98.0834) -> (-112.8683, -98.0834)
  line L59 (-112.8683, -98.0834) -> (-112.8683, -103.8834)
  line L60 (-112.8683, -103.8834) -> (-112.0689, -103.8834)
  line L61 (-112.0689, -103.8834) -> (-112.0689, -106.9826)
  line L62 (-112.0689, -106.9826) -> (-112.8683, -106.9826)
  line L63 (-112.8683, -106.9826) -> (-112.8683, -107.9831)
  line L64 (-170.02, -107.9831) -> (-184.019, -107.9831)
  line L65 (-184.019, -107.9831) -> (-184.019, -106.9826)
  line L66 (-184.019, -106.9826) -> (-184.82, -106.9826)
  line L67 (-184.82, -106.9826) -> (-184.82, -103.8834)
  line L68 (-184.82, -103.8834) -> (-184.019, -103.8834)
  line L69 (-184.019, -103.8834) -> (-184.019, -98.0834)
  line L70 (-184.019, -98.0834) -> (-184.82, -98.0834)
  line L71 (-184.82, -98.0834) -> (-184.82, -94.9828)
  line L72 (-184.82, -94.9828) -> (-184.019, -94.9828)
  line L73 (-184.019, -94.9828) -> (-184.019, -93.9838)
  line L74 (-184.019, -93.9838) -> (-170.02, -93.9838)
  line L75 (-170.02, -93.9838) -> (-170.02, -94.9828)
  line L76 (-170.02, -94.9828) -> (-169.219, -94.9828)
  line L77 (-169.219, -94.9828) -> (-169.219, -98.0834)
  line L78 (-169.219, -98.0834) -> (-170.02, -98.0834)
  line L79 (-170.02, -98.0834) -> (-170.02, -103.8834)
  line L80 (-170.02, -103.8834) -> (-169.219, -103.8834)
  line L81 (-169.219, -103.8834) -> (-169.219, -106.9826)
  line L82 (-169.219, -106.9826) -> (-170.02, -106.9826)
  line L83 (-170.02, -106.9826) -> (-170.02, -107.9831)
  line L84 (-24.762, -69.8831) -> (-38.7629, -69.8831)
  line L85 (-38.7629, -69.8831) -> (-38.7629, -68.8826)
  line L86 (-38.7629, -68.8826) -> (-39.5622, -68.8826)
  line L87 (-39.5622, -68.8826) -> (-39.5622, -65.7834)
  line L88 (-39.5622, -65.7834) -> (-38.7629, -65.7834)
  line L89 (-38.7629, -65.7834) -> (-38.7629, -59.9834)
  line L90 (-38.7629, -59.9834) -> (-39.5622, -59.9834)
  line L91 (-39.5622, -59.9834) -> (-39.5622, -56.8828)
  line L92 (-39.5622, -56.8828) -> (-38.7629, -56.8828)
  line L93 (-38.7629, -56.8828) -> (-38.7629, -55.8838)
  line L94 (-38.7629, -55.8838) -> (-24.762, -55.8838)
  line L95 (-24.762, -55.8838) -> (-24.762, -56.8828)
  line L96 (-24.762, -56.8828) -> (-23.9628, -56.8828)
  line L97 (-23.9628, -56.8828) -> (-23.9628, -59.9834)
  line L98 (-23.9628, -59.9834) -> (-24.762, -59.9834)
  line L99 (-24.762, -59.9834) -> (-24.762, -65.7834)
  line L100 (-24.762, -65.7834) -> (-23.9628, -65.7834)
  line L101 (-23.9628, -65.7834) -> (-23.9628, -68.8826)
  line L102 (-23.9628, -68.8826) -> (-24.762, -68.8826)
  line L103 (-24.762, -68.8826) -> (-24.762, -69.8831)
  line L104 (-93.8197, -107.9831) -> (-107.819, -107.9831)
  line L105 (-107.819, -107.9831) -> (-107.819, -106.9826)
  line L106 (-107.819, -106.9826) -> (-108.6184, -106.9826)
  line L107 (-108.6184, -106.9826) -> (-108.6184, -103.8834)
  line L108 (-108.6184, -103.8834) -> (-107.819, -103.8834)
  line L109 (-107.819, -103.8834) -> (-107.819, -98.0834)
  line L110 (-107.819, -98.0834) -> (-108.6184, -98.0834)
  line L111 (-108.6184, -98.0834) -> (-108.6184, -94.9828)
  line L112 (-108.6184, -94.9828) -> (-107.819, -94.9828)
  line L113 (-107.819, -94.9828) -> (-107.819, -93.9838)
  line L114 (-107.819, -93.9838) -> (-93.8197, -93.9838)
  line L115 (-93.8197, -93.9838) -> (-93.8197, -94.9828)
  line L116 (-93.8197, -94.9828) -> (-93.0189, -94.9828)
  line L117 (-93.0189, -94.9828) -> (-93.0189, -98.0834)
  line L118 (-93.0189, -98.0834) -> (-93.8197, -98.0834)
  line L119 (-93.8197, -98.0834) -> (-93.8197, -103.8834)
  line L120 (-93.8197, -103.8834) -> (-93.0189, -103.8834)
  line L121 (-93.0189, -103.8834) -> (-93.0189, -106.9826)
  line L122 (-93.0189, -106.9826) -> (-93.8197, -106.9826)
  line L123 (-93.8197, -106.9826) -> (-93.8197, -107.9831)
  line L124 (-55.7197, -107.9831) -> (-69.719, -107.9831)
  line L125 (-69.719, -107.9831) -> (-69.719, -106.9826)
  line L126 (-69.719, -106.9826) -> (-70.5198, -106.9826)
  line L127 (-70.5198, -106.9826) -> (-70.5198, -103.8834)
  line L128 (-70.5198, -103.8834) -> (-69.719, -103.8834)
  line L129 (-69.719, -103.8834) -> (-69.719, -98.0834)
  line L130 (-69.719, -98.0834) -> (-70.5198, -98.0834)
  line L131 (-70.5198, -98.0834) -> (-70.5198, -94.9828)
  line L132 (-70.5198, -94.9828) -> (-69.719, -94.9828)
  line L133 (-69.719, -94.9828) -> (-69.719, -93.9838)
  line L134 (-69.719, -93.9838) -> (-55.7197, -93.9838)
  line L135 (-55.7197, -93.9838) -> (-55.7197, -94.9828)
  line L136 (-55.7197, -94.9828) -> (-54.9189, -94.9828)
  line L137 (-54.9189, -94.9828) -> (-54.9189, -98.0834)
  line L138 (-54.9189, -98.0834) -> (-55.7197, -98.0834)
  line L139 (-55.7197, -98.0834) -> (-55.7197, -103.8834)
  line L140 (-55.7197, -103.8834) -> (-54.9189, -103.8834)
  line L141 (-54.9189, -103.8834) -> (-54.9189, -106.9826)
  line L142 (-54.9189, -106.9826) -> (-55.7197, -106.9826)
  line L143 (-55.7197, -106.9826) -> (-55.7197, -107.9831)
  line L144 (-258.126, -31.7831) -> (-272.125, -31.7831)
  line L145 (-272.125, -31.7831) -> (-272.125, -30.7827)
  line L146 (-272.125, -30.7827) -> (-272.926, -30.7827)
  line L147 (-272.926, -30.7827) -> (-272.926, -27.6848)
  line L148 (-272.926, -27.6848) -> (-272.125, -27.6848)
  line L149 (-272.125, -27.6848) -> (-272.125, -21.8833)
  line L150 (-272.125, -21.8833) -> (-272.926, -21.8833)
  line L151 (-272.926, -21.8833) -> (-272.926, -18.7827)
  line L152 (-272.926, -18.7827) -> (-272.125, -18.7827)
  line L153 (-272.125, -18.7827) -> (-272.125, -17.7836)
  line L154 (-272.125, -17.7836) -> (-258.126, -17.7836)
  line L155 (-258.126, -17.7836) -> (-258.126, -18.7827)
  line L156 (-258.126, -18.7827) -> (-257.325, -18.7827)
  line L157 (-257.325, -18.7827) -> (-257.325, -21.8833)
  line L158 (-257.325, -21.8833) -> (-258.126, -21.8833)
  line L159 (-258.126, -21.8833) -> (-258.126, -27.6848)
  line L160 (-258.126, -27.6848) -> (-257.325, -27.6848)
  line L161 (-257.325, -27.6848) -> (-257.325, -30.7827)
  line L162 (-257.325, -30.7827) -> (-258.126, -30.7827)
  line L163 (-258.126, -30.7827) -> (-258.126, -31.7831)
  line L164 (-210.501, -31.7831) -> (-224.5, -31.7831)
  line L165 (-224.5, -31.7831) -> (-224.5, -30.7827)
  line L166 (-224.5, -30.7827) -> (-225.301, -30.7827)
  line L167 (-225.301, -30.7827) -> (-225.301, -27.6848)
  line L168 (-225.301, -27.6848) -> (-224.5, -27.6848)
  line L169 (-224.5, -27.6848) -> (-224.5, -21.8833)
  line L170 (-224.5, -21.8833) -> (-225.301, -21.8833)
  line L171 (-225.301, -21.8833) -> (-225.301, -18.7827)
  line L172 (-225.301, -18.7827) -> (-224.5, -18.7827)
  line L173 (-224.5, -18.7827) -> (-224.5, -17.7836)
  line L174 (-224.5, -17.7836) -> (-210.501, -17.7836)
  line L175 (-210.501, -17.7836) -> (-210.501, -18.7827)
  line L176 (-210.501, -18.7827) -> (-209.7, -18.7827)
  line L177 (-209.7, -18.7827) -> (-209.7, -21.8833)
  line L178 (-209.7, -21.8833) -> (-210.501, -21.8833)
  line L179 (-210.501, -21.8833) -> (-210.501, -27.6848)
  line L180 (-210.501, -27.6848) -> (-209.7, -27.6848)
  line L181 (-209.7, -27.6848) -> (-209.7, -30.7827)
  line L182 (-209.7, -30.7827) -> (-210.501, -30.7827)
  line L183 (-210.501, -30.7827) -> (-210.501, -31.7831)
  line L184 (-150.97, -107.9831) -> (-164.969, -107.9831)
  line L185 (-164.969, -107.9831) -> (-164.969, -106.9826)
  line L186 (-164.969, -106.9826) -> (-165.77, -106.9826)
  line L187 (-165.77, -106.9826) -> (-165.77, -103.8834)
  line L188 (-165.77, -103.8834) -> (-164.969, -103.8834)
  line L189 (-164.969, -103.8834) -> (-164.969, -98.0834)
  line L190 (-164.969, -98.0834) -> (-165.77, -98.0834)
  line L191 (-165.77, -98.0834) -> (-165.77, -94.9828)
  line L192 (-165.77, -94.9828) -> (-164.969, -94.9828)
  line L193 (-164.969, -94.9828) -> (-164.969, -93.9838)
  line L194 (-164.969, -93.9838) -> (-150.97, -93.9838)
  line L195 (-150.97, -93.9838) -> (-150.97, -94.9828)
  line L196 (-150.97, -94.9828) -> (-150.169, -94.9828)
  line L197 (-150.169, -94.9828) -> (-150.169, -98.0834)
  line L198 (-150.169, -98.0834) -> (-150.97, -98.0834)
  line L199 (-150.97, -98.0834) -> (-150.97, -103.8834)
  line L200 (-150.97, -103.8834) -> (-150.169, -103.8834)
  line L201 (-150.169, -103.8834) -> (-150.169, -106.9826)
  line L202 (-150.169, -106.9826) -> (-150.97, -106.9826)
  line L203 (-150.97, -106.9826) -> (-150.97, -107.9831)
  line L204 (-131.918, -107.9831) -> (-145.919, -107.9831)
  line L205 (-145.919, -107.9831) -> (-145.919, -106.9826)
  line L206 (-145.919, -106.9826) -> (-146.72, -106.9826)
  line L207 (-146.72, -106.9826) -> (-146.72, -103.8834)
  line L208 (-146.72, -103.8834) -> (-145.919, -103.8834)
  line L209 (-145.919, -103.8834) -> (-145.919, -98.0834)
  line L210 (-145.919, -98.0834) -> (-146.72, -98.0834)
  line L211 (-146.72, -98.0834) -> (-146.72, -94.9828)
  line L212 (-146.72, -94.9828) -> (-145.919, -94.9828)
  line L213 (-145.919, -94.9828) -> (-145.919, -93.9838)
  line L214 (-145.919, -93.9838) -> (-131.918, -93.9838)
  line L215 (-131.918, -93.9838) -> (-131.918, -94.9828)
  line L216 (-131.918, -94.9828) -> (-131.119, -94.9828)
  line L217 (-131.119, -94.9828) -> (-131.119, -98.0834)
  line L218 (-131.119, -98.0834) -> (-131.918, -98.0834)
  line L219 (-131.918, -98.0834) -> (-131.918, -103.8834)
  line L220 (-131.918, -103.8834) -> (-131.119, -103.8834)
  line L221 (-131.119, -103.8834) -> (-131.119, -106.9826)
  line L222 (-131.119, -106.9826) -> (-131.918, -106.9826)
  line L223 (-131.918, -106.9826) -> (-131.918, -107.9831)
  line L224 (-22.3822, -88.9331) -> (-36.3817, -88.9331)
  line L225 (-36.3817, -88.9331) -> (-36.3817, -87.9326)
  line L226 (-36.3817, -87.9326) -> (-37.1809, -87.9326)
  line L227 (-37.1809, -87.9326) -> (-37.1809, -84.8334)
  line L228 (-37.1809, -84.8334) -> (-36.3817, -84.8334)
  line L229 (-36.3817, -84.8334) -> (-36.3817, -79.0334)
  line L230 (-36.3817, -79.0334) -> (-37.1809, -79.0334)
  line L231 (-37.1809, -79.0334) -> (-37.1809, -75.9328)
  line L232 (-37.1809, -75.9328) -> (-36.3817, -75.9328)
  line L233 (-36.3817, -75.9328) -> (-36.3817, -74.9338)
  line L234 (-36.3817, -74.9338) -> (-22.3822, -74.9338)
  line L235 (-22.3822, -74.9338) -> (-22.3822, -75.9328)
  line L236 (-22.3822, -75.9328) -> (-21.5815, -75.9328)
  line L237 (-21.5815, -75.9328) -> (-21.5815, -79.0334)
  line L238 (-21.5815, -79.0334) -> (-22.3822, -79.0334)
  line L239 (-22.3822, -79.0334) -> (-22.3822, -84.8334)
  line L240 (-22.3822, -84.8334) -> (-21.5815, -84.8334)
  line L241 (-21.5815, -84.8334) -> (-21.5815, -87.9326)
  line L242 (-21.5815, -87.9326) -> (-22.3822, -87.9326)
  line L243 (-22.3822, -87.9326) -> (-22.3822, -88.9331)
  line L244 (-50.9572, -69.8831) -> (-64.9565, -69.8831)
  line L245 (-64.9565, -69.8831) -> (-64.9565, -68.8826)
  line L246 (-64.9565, -68.8826) -> (-65.7559, -68.8826)
  line L247 (-65.7559, -68.8826) -> (-65.7559, -65.7834)
  line L248 (-65.7559, -65.7834) -> (-64.9565, -65.7834)
  line L249 (-64.9565, -65.7834) -> (-64.9565, -59.9834)
  line L250 (-64.9565, -59.9834) -> (-65.7559, -59.9834)
  line L251 (-65.7559, -59.9834) -> (-65.7559, -56.8828)
  line L252 (-65.7559, -56.8828) -> (-64.9565, -56.8828)
  line L253 (-64.9565, -56.8828) -> (-64.9565, -55.8838)
  line L254 (-64.9565, -55.8838) -> (-50.9572, -55.8838)
  line L255 (-50.9572, -55.8838) -> (-50.9572, -56.8828)
  line L256 (-50.9572, -56.8828) -> (-50.1565, -56.8828)
  line L257 (-50.1565, -56.8828) -> (-50.1565, -59.9834)
  line L258 (-50.1565, -59.9834) -> (-50.9572, -59.9834)
  line L259 (-50.9572, -59.9834) -> (-50.9572, -65.7834)
  line L260 (-50.9572, -65.7834) -> (-50.1565, -65.7834)
  line L261 (-50.1565, -65.7834) -> (-50.1565, -68.8826)
  line L262 (-50.1565, -68.8826) -> (-50.9572, -68.8826)
  line L263 (-50.9572, -68.8826) -> (-50.9572, -69.8831)
  line L264 (-146.207, -69.8831) -> (-160.207, -69.8831)
  line L265 (-160.207, -69.8831) -> (-160.207, -68.8826)
  line L266 (-160.207, -68.8826) -> (-161.006, -68.8826)
  line L267 (-161.006, -68.8826) -> (-161.006, -65.7834)
  line L268 (-161.006, -65.7834) -> (-160.207, -65.7834)
  line L269 (-160.207, -65.7834) -> (-160.207, -59.9834)
  line L270 (-160.207, -59.9834) -> (-161.006, -59.9834)
  line L271 (-161.006, -59.9834) -> (-161.006, -56.8828)
  line L272 (-161.006, -56.8828) -> (-160.207, -56.8828)
  line L273 (-160.207, -56.8828) -> (-160.207, -55.8838)
  line L274 (-160.207, -55.8838) -> (-146.207, -55.8838)
  line L275 (-146.207, -55.8838) -> (-146.207, -56.8828)
  line L276 (-146.207, -56.8828) -> (-145.406, -56.8828)
  line L277 (-145.406, -56.8828) -> (-145.406, -59.9834)
  line L278 (-145.406, -59.9834) -> (-146.207, -59.9834)
  line L279 (-146.207, -59.9834) -> (-146.207, -65.7834)
  line L280 (-146.207, -65.7834) -> (-145.406, -65.7834)
  line L281 (-145.406, -65.7834) -> (-145.406, -68.8826)
  line L282 (-145.406, -68.8826) -> (-146.207, -68.8826)
  line L283 (-146.207, -68.8826) -> (-146.207, -69.8831)
  line L284 (-155.732, -50.833) -> (-169.732, -50.833)
  line L285 (-169.732, -50.833) -> (-169.732, -49.8327)
  line L286 (-169.732, -49.8327) -> (-170.531, -49.8327)
  line L287 (-170.531, -49.8327) -> (-170.531, -46.7348)
  line L288 (-170.531, -46.7348) -> (-169.732, -46.7348)
  line L289 (-169.732, -46.7348) -> (-169.732, -40.9333)
  line L290 (-169.732, -40.9333) -> (-170.531, -40.9333)
  line L291 (-170.531, -40.9333) -> (-170.531, -37.8327)
  line L292 (-170.531, -37.8327) -> (-169.732, -37.8327)
  line L293 (-169.732, -37.8327) -> (-169.732, -36.8336)
  line L294 (-169.732, -36.8336) -> (-155.732, -36.8336)
  line L295 (-155.732, -36.8336) -> (-155.732, -37.8327)
  line L296 (-155.732, -37.8327) -> (-154.931, -37.8327)
  line L297 (-154.931, -37.8327) -> (-154.931, -40.9333)
  line L298 (-154.931, -40.9333) -> (-155.732, -40.9333)
  line L299 (-155.732, -40.9333) -> (-155.732, -46.7348)
  line L300 (-155.732, -46.7348) -> (-154.931, -46.7348)
  line L301 (-154.931, -46.7348) -> (-154.931, -49.8327)
  line L302 (-154.931, -49.8327) -> (-155.732, -49.8327)
  line L303 (-155.732, -49.8327) -> (-155.732, -50.833)
  line L304 (-174.782, -50.833) -> (-188.782, -50.833)
  line L305 (-188.782, -50.833) -> (-188.782, -49.8327)
  line L306 (-188.782, -49.8327) -> (-189.581, -49.8327)
  line L307 (-189.581, -49.8327) -> (-189.581, -46.7348)
  line L308 (-189.581, -46.7348) -> (-188.782, -46.7348)
  line L309 (-188.782, -46.7348) -> (-188.782, -40.9333)
  line L310 (-188.782, -40.9333) -> (-189.581, -40.9333)
  line L311 (-189.581, -40.9333) -> (-189.581, -37.8327)
  line L312 (-189.581, -37.8327) -> (-188.782, -37.8327)
  line L313 (-188.782, -37.8327) -> (-188.782, -36.8336)
  line L314 (-188.782, -36.8336) -> (-174.782, -36.8336)
  line L315 (-174.782, -36.8336) -> (-174.782, -37.8327)
  line L316 (-174.782, -37.8327) -> (-173.981, -37.8327)
  line L317 (-173.981, -37.8327) -> (-173.981, -40.9333)
  line L318 (-173.981, -40.9333) -> (-174.782, -40.9333)
  line L319 (-174.782, -40.9333) -> (-174.782, -46.7348)
  line L320 (-174.782, -46.7348) -> (-173.981, -46.7348)
  line L321 (-173.981, -46.7348) -> (-173.981, -49.8327)
  line L322 (-173.981, -49.8327) -> (-174.782, -49.8327)
  line L323 (-174.782, -49.8327) -> (-174.782, -50.833)
  line L324 (-179.545, -88.9331) -> (-193.544, -88.9331)
  line L325 (-193.544, -88.9331) -> (-193.544, -87.9326)
  line L326 (-193.544, -87.9326) -> (-194.345, -87.9326)
  line L327 (-194.345, -87.9326) -> (-194.345, -84.8334)
  line L328 (-194.345, -84.8334) -> (-193.544, -84.8334)
  line L329 (-193.544, -84.8334) -> (-193.544, -79.0334)
  line L330 (-193.544, -79.0334) -> (-194.345, -79.0334)
  line L331 (-194.345, -79.0334) -> (-194.345, -75.9328)
  line L332 (-194.345, -75.9328) -> (-193.544, -75.9328)
  line L333 (-193.544, -75.9328) -> (-193.544, -74.9338)
  line L334 (-193.544, -74.9338) -> (-179.545, -74.9338)
  line L335 (-179.545, -74.9338) -> (-179.545, -75.9328)
  line L336 (-179.545, -75.9328) -> (-178.744, -75.9328)
  line L337 (-178.744, -75.9328) -> (-178.744, -79.0334)
  line L338 (-178.744, -79.0334) -> (-179.545, -79.0334)
  line L339 (-179.545, -79.0334) -> (-179.545, -84.8334)
  line L340 (-179.545, -84.8334) -> (-178.744, -84.8334)
  line L341 (-178.744, -84.8334) -> (-178.744, -87.9326)
  line L342 (-178.744, -87.9326) -> (-179.545, -87.9326)
  line L343 (-179.545, -87.9326) -> (-179.545, -88.9331)
  line L344 (-79.5322, -50.833) -> (-93.5315, -50.833)
  line L345 (-93.5315, -50.833) -> (-93.5315, -49.8327)
  line L346 (-93.5315, -49.8327) -> (-94.3309, -49.8327)
  line L347 (-94.3309, -49.8327) -> (-94.3309, -46.7348)
  line L348 (-94.3309, -46.7348) -> (-93.5315, -46.7348)